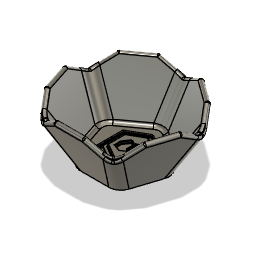
GB - Porta D12 (Autodesk Fusion 360 design; units mm, degrees)
Autodesk Fusion 360 part; units mm, degrees
note: some values were not read from the file. Chosen so that the rebuilt part matches the saved one: which bodies a step acts on; which face or edge a step refers to. Set by a fixed rule: which sketch regions a step uses.
sketch "Sketch1" plane through (0, 0, 0) normal (0, 1, 0) x (1, 0, 0)
  line L0 (-5, -6.8819) -> (5, -6.8819)
  line L1 (5, -6.8819) -> (8.0902, 2.6287)
  line L2 (8.0902, 2.6287) -> (0, 8.5065)
  line L3 (0, 8.5065) -> (-8.0902, 2.6287)
  line L4 (-8.0902, 2.6287) -> (-5, -6.8819)
  dimension "d1" = 10
  constraint horizontal L0
  measures "d1" distance of L0.start L0.end
ref_plane "WorkPlane1" through (0, 0, 6.8819) normal (0, -0.447213, 0.894428) x (1, 0, 0)
ref_plane "WorkPlane2" through (-6.5451, 0, 2.1266) normal (-0.850651, -0.447213, 0.276393) x (0.309017, 0, 0.951057)
ref_plane "WorkPlane3" through (-4.0451, 0, -5.5676) normal (0.525731, 0.447213, 0.723607) x (-0.809017, 0, 0.587785)
ref_plane "WorkPlane4" through (4.0451, 0, -5.5676) normal (-0.525731, 0.447213, 0.723607) x (-0.809017, 0, -0.587785)
ref_plane "WorkPlane5" through (6.5451, 0, 2.1266) normal (0.850651, -0.447213, 0.276393) x (0.309017, 0, -0.951057)
sketch "Sketch2" plane through (15, -2.7528, 5.5055) normal (0, -0.447213, 0.894428) x (1, 0, 0)
  line L0 (-10, 3.0777) -> (-6.9098, 12.5882)
  line L1 (-6.9098, 12.5882) -> (-15, 18.4661)
  line L2 (-15, 18.4661) -> (-23.0902, 12.5882)
  line L3 (-23.0902, 12.5882) -> (-20, 3.0777)
  line L4 (-20, 3.0777) -> (-10, 3.0777)
  point P0 (-15, 9.9596)
  point P1 (-10, 3.0777)
  point P2 (-20, 3.0777)
  constraint coincident L0.start L4.end
  constraint coincident P2 L3.end
sketch "Sketch3" plane through (18.1631, 8.6599, -19.618) normal (0.850651, -0.447213, 0.276393) x (0.309017, 0, -0.951057)
  line L0 (-19.2705, -9.6821) -> (-16.1803, -0.1715)
  line L1 (-16.1803, -0.1715) -> (-24.2705, 5.7064)
  line L2 (-24.2705, 5.7064) -> (-32.3607, -0.1715)
  line L3 (-32.3607, -0.1715) -> (-29.2705, -9.6821)
  line L4 (-29.2705, -9.6821) -> (-19.2705, -9.6821)
  point P0 (-24.2705, -2.8002)
  point P1 (-19.2705, -9.6821)
  point P2 (-29.2705, -9.6821)
  constraint coincident P2 L3.end
  constraint coincident L0.start L4.end
sketch "Sketch4" plane through (8.6631, 15.7133, -11.9237) normal (-0.525731, 0.447213, 0.723607) x (-0.809017, 0, -0.587785)
  line L0 (5, 17.568) -> (-5, 17.568)
  line L1 (-5, 17.568) -> (-8.0902, 8.0574)
  line L2 (-8.0902, 8.0574) -> (0, 2.1796)
  line L3 (0, 2.1796) -> (8.0902, 8.0574)
  line L4 (8.0902, 8.0574) -> (5, 17.568)
  point P0 (0, 10.6861)
  point P1 (5, 17.568)
  point P2 (-5, 17.568)
  constraint coincident L0.end L1.start
  constraint coincident L0.start L4.end
sketch "Sketch5" plane through (13.0451, 8.6599, -23.3364) normal (0.525731, 0.447213, 0.723607) x (-0.809017, 0, 0.587785)
  line L0 (29.2705, 9.6821) -> (19.2705, 9.6821)
  line L1 (19.2705, 9.6821) -> (16.1803, 0.1715)
  line L2 (16.1803, 0.1715) -> (24.2705, -5.7064)
  line L3 (24.2705, -5.7064) -> (32.3607, 0.1715)
  line L4 (32.3607, 0.1715) -> (29.2705, 9.6821)
  point P0 (24.2705, 2.8002)
  point P1 (29.2705, 9.6821)
  point P2 (19.2705, 9.6821)
  constraint coincident L0.end L1.start
  constraint coincident L0.start L4.end
sketch "Sketch6" plane through (-9.8713, -2.7528, -12.5645) normal (-0.850651, -0.447213, 0.276393) x (0.309017, 0, 0.951057)
  line L0 (20, 3.0777) -> (23.0902, 12.5882)
  line L1 (23.0902, 12.5882) -> (15, 18.4661)
  line L2 (15, 18.4661) -> (6.9098, 12.5882)
  line L3 (6.9098, 12.5882) -> (10, 3.0777)
  line L4 (10, 3.0777) -> (20, 3.0777)
  point P0 (15, 9.9596)
  point P1 (10, 3.0777)
  point P2 (20, 3.0777)
  constraint coincident P1 L3.end
  constraint coincident P2 L0.start
extrude "Extrude2" add sketch "Sketch1" along normal blind 2 makes body 1
extrude "Extrude3" add sketch "Sketch6" against normal blind 1 bodies 1
extrude "Extrude4" add sketch "Sketch2" against normal blind 1 bodies 1
extrude "Extrude5" add sketch "Sketch3" against normal blind 1 bodies 1
extrude "Extrude6" add sketch "Sketch4" along normal blind 1 bodies 1
extrude "Extrude7" add sketch "Sketch5" along normal blind 1 bodies 1
ref_plane "WorkPlane9" through (0, 12, 0) normal (0, 1, 0) x (0, 0, 1)
split "Split1" by plane through (0, 12, 0) normal (0, 1, 0) bodies 1 makes body 2 at (-7.1312, 12.737, -9.8153) makes body 3 at (-11.5386, 12.737, 3.7491) makes body 4 at (0, 12.737, 12.1324) makes body 5 at (7.1312, 12.737, -9.8153) makes body 6 at (11.5386, 12.737, 3.7491)
delete_body "RemoveBody1" bodies 5
delete_body "RemoveBody2" bodies 4
delete_body "RemoveBody3" bodies 6
delete_body "RemoveBody4" bodies 3
delete_body "RemoveBody5" bodies 2
fillet "Fillet2" radius 3 10 edges at (-6.5451, 4.2533, 9.0085) (-10.5902, 4.2533, -3.441) (0, 4.2533, -11.1352) (10.5902, 4.2533, -3.441) (6.5451, 4.2533, 9.0085) (0, 5.6477, -10.615) (6.2393, 5.6477, 8.5877) (-6.2393, 5.6477, 8.5877) (10.0955, 5.6477, -3.2802) (-10.0955, 5.6477, -3.2802) on bodies 1
fillet "Fillet6" radius 1 10 edges at (-3.9757, 2, -5.4721) (-7.3625, 2, -2.3922) (0, 2, -7.7414) (-6.4328, 2, 2.0902) (3.9757, 2, -5.4721) (-4.5503, 2, 6.2629) (7.3625, 2, -2.3922) (0, 2, 6.7639) (6.4328, 2, 2.0902) (4.5503, 2, 6.2629) on bodies 1
sketch "Sketch8" plane through (0, 2, 0) normal (0, 1, 0) x (-1, 0, 0)
  line L0 (0, -4.7528) -> (3.25, -2.8764)
  line L1 (3.25, -2.8764) -> (3.25, 0.8764)
  line L2 (3.25, 0.8764) -> (0, 2.7528)
  line L3 (0, 2.7528) -> (-3.25, 0.8764)
  line L4 (-3.25, 0.8764) -> (-3.25, -2.8764)
  line L5 (-3.25, -2.8764) -> (0, -4.7528)
  line L6 (0, 0) -> (0, -1)
  line L7 (0, 3.6188) -> (-3.25, 1.7424)
  line L8 (-4, 1.3094) -> (-4, -3.3094)
  line L9 (-4, -3.3094) -> (0, -5.6188)
  line L10 (0, -5.6188) -> (4, -3.3094)
  line L11 (4, -3.3094) -> (4, 1.3094)
  line L12 (3.25, 1.7424) -> (0, 3.6188)
  line L13 (-4, 1.3094) -> (-4, 2.3094)
  line L14 (4, 1.3094) -> (4, 2.3094)
  line L15 (-3.25, 2.7424) -> (0, 4.6188)
  line L16 (0, 3.6188) -> (0, 4.6188)
  line L17 (-4, 2.3094) -> (-4, 3.0594)
  line L18 (0, 4.6188) -> (0, 5.3688)
  line L19 (-4, 3.0594) -> (0, 5.3688)
  line L20 (-3.25, 1.7424) -> (-3.25, 2.7424)
  line L21 (4, 2.3094) -> (0, 4.6188)
  line L22 (3.25, 1.7424) -> (3.25, 2.7424)
  line L23 (0, 5.3688) -> (4, 3.0594)
  line L24 (4, 3.0594) -> (4, 2.3094)
  line L25 (0, 0) -> (0, 3.6188)
  line L26 (0, 4.6188) -> (0, 5.3688)
  line L27 (0, 3.6188) -> (0, 4.6188)
  line L28 (-3.25, 1.7424) -> (-4, 1.3094)
  line L29 (-4, 2.3094) -> (-3.25, 2.7424)
  line L30 (4, 1.3094) -> (3.25, 1.7424)
  point P0 (0, -1)
  point P1 (0, -1)
  dimension "d35" = 1
  dimension "d37" = 1
  dimension "d40" = 0.75
  dimension "d43" = 3.25
  dimension "d44" = 4
  constraint coincident L6.start L25.start
  constraint coincident P1 P0
  constraint parallel L8 L13
  constraint parallel L11 L14
  constraint parallel L13 L17
  constraint parallel L16 L18
  constraint collinear L4 L20
  constraint coincident L21 L22.end
  constraint parallel L6 L25
  constraint collinear L1 L22
  constraint collinear L11 L24
  constraint vertical L25
  constraint parallel L2 L12
  constraint parallel L12 L21
  constraint equal L13 L14
  constraint equal L17 L24
  constraint vertical L11
  constraint parallel L2 L30
  constraint equal L13 L27
  constraint equal L17 L18
  measures "d35" distance of L6.start P1
  measures "d37" distance of L8.start L13.end
  measures "d40" distance of L13.end L17.end
  measures "d43" distance of P1 L4
  measures "d44" distance of P1 L8
sketch "Sketch9" plane through (0, 2, 0) normal (0, 1, 0) x (-1, 0, 0)
  line L0 (3.1655, 6.1458) -> (-3.1655, 6.1458)
  line L1 (-4.8668, 4.9098) -> (-6.8232, -1.1114)
  line L2 (-6.1734, -3.1114) -> (-1.0515, -6.8327)
  line L3 (1.0515, -6.8327) -> (6.1734, -3.1114)
  line L4 (6.8232, -1.1114) -> (4.8668, 4.9098)
  ellipse E0 centre (4.5962, -1.4934) end of major axis (6.8323, -2.2199) minor radius 2 (6.1734, -3.1114) -> (6.8232, -1.1114) ccw construction
  ellipse E1 centre (2.8406, 3.9098) end of major axis (4.2226, 5.8119) minor radius 2 (4.8668, 4.9098) -> (3.1655, 6.1458) ccw construction
  ellipse E2 centre (-2.8406, 3.9098) end of major axis (-4.2226, 5.8119) minor radius 2 (-3.1655, 6.1458) -> (-4.8668, 4.9098) ccw construction
  ellipse E3 centre (-4.5962, -1.4934) end of major axis (-6.8323, -2.2199) minor radius 2 (-6.8232, -1.1114) -> (-6.1734, -3.1114) ccw construction
  ellipse E4 centre (0, -4.8327) end of major axis (0, -7.1839) minor radius 2 (-1.0515, -6.8327) -> (1.0515, -6.8327) ccw construction
  line L5 (-2.5118, -0.3911) -> (-2.3485, -1.8376)
  line L6 (-2.3485, -1.8376) -> (-1.4619, -2.8642)
  line L7 (-1.4619, -2.8642) -> (0.0888, -2.1176)
  line L8 (0.0888, -2.1176) -> (0.0888, -0.5078)
  line L9 (0.0888, -0.5078) -> (-0.8554, 0.3088)
  line L10 (-0.8554, 0.3088) -> (-2.5118, -0.3911)
  line L11 (0.3403, -1.9543) -> (1.2969, -2.4428)
  line L12 (1.2969, -2.4428) -> (2.2301, -1.0662)
  line L13 (2.2301, -1.0662) -> (2.2301, 0.217)
  line L14 (2.2301, 0.217) -> (0.7836, 0.7535)
  line L15 (0.7836, 0.7535) -> (-0.213, 0.045)
  line L16 (-0.213, 0.045) -> (0.3403, -0.413)
  line L17 (0.3403, -0.413) -> (0.3403, -1.9543)
extrude "Extrude8" cut sketch "Sketch8" sketch "Sketch9" against normal blind 0.5 contours L7 L8 L9 L10 L11 L12 L28 L30 | L13 L20 L28 L29 | L14 L21 L22 L30 | L15 L17 L18 L19 L26 L29 | L18 L21 L23 L24 L26 of sketch 2 bodies 1
fillet "Fillet8" radius 0.1 31 edges at (2, 1.5, -4.4641) (-2, 1.5, -4.4641) (-4, 1.5, -0.125) (-2, 1.5, 4.2141) (2, 1.5, 4.2141) (4, 1.5, -0.125) (1.625, 1.5, 3.6806) (-1.625, 1.5, 3.6806) (-3.25, 1.5, 2.2424) (-1.625, 1.5, 2.6806) (1.625, 1.5, 2.6806) (3.25, 1.5, 2.2424) (1.625, 1.5, -3.8146) (3.25, 1.5, -1) (1.625, 1.5, 1.8146) (-1.625, 1.5, 1.8146) (-3.25, 1.5, -1) (-1.625, 1.5, -3.8146) (-0.3403, 1.5, -1.1836) (-0.8186, 1.5, -2.1985) (-1.7635, 1.5, -1.7545) (-2.2301, 1.5, -0.4246) (-1.5069, 1.5, 0.4852) (-0.2853, 1.5, 0.3993) (-0.0637, 1.5, -0.184) (1.6836, 1.5, -0.0412) (2.4301, 1.5, -1.1144) (1.9052, 1.5, -2.3509) (0.6866, 1.5, -2.4909) (-0.0888, 1.5, -1.3127) (0.3833, 1.5, -0.0995) on bodies 1
fillet "Fillet9" radius 0.15 18 edges at (2, 2, 4.2141) (4, 2, -0.125) (1.625, 2, 3.6806) (1.625, 2, 2.6806) (3.25, 2, 2.2424) (-1.625, 2, 2.6806) (-1.625, 2, 3.6806) (-2, 2, 4.2141) (-4, 2, -0.125) (-1.625, 2, 1.8146) (-3.25, 2, 2.2424) (-2, 2, -4.4641) (-1.625, 2, -3.8146) (2, 2, -4.4641) (1.625, 2, -3.8146) (3.25, 2, -1) (-3.25, 2, -1) (1.625, 2, 1.8146) on bodies 1
fillet "Fillet10" radius 0.1 13 edges at (0.6866, 2, -2.4909) (1.9052, 2, -2.3509) (2.4301, 2, -1.1144) (1.6836, 2, -0.0412) (0.3833, 2, -0.0995) (-0.2853, 2, 0.3993) (-0.3403, 2, -1.1836) (-1.5069, 2, 0.4852) (-0.0637, 2, -0.184) (-2.2301, 2, -0.4246) (-1.7635, 2, -1.7545) (-0.8186, 2, -2.1985) (-0.0888, 2, -1.3127) on bodies 1
fillet "Fillet12" radius 0.5 65 edges at (-10.466, 11.1601, -6.4179) (-6.9146, 12, -9.5172) (-2.8696, 11.1601, -11.937) (-11.6357, 9.9182, -4.6427) (-12.1424, 9.9182, -3.0833) (0.8198, 9.9182, -12.5009) (-0.8198, 9.9182, -12.5009) (-12.2395, 11.1601, -0.9596) (-11.1881, 12, 3.6352) (-9.3379, 11.1601, 7.9705) (10.466, 11.1601, -6.4179) (6.9146, 12, -9.5172) (2.8696, 11.1601, -11.937) (-6.6846, 9.9182, 10.5953) (-8.0111, 9.9182, 9.6316) (12.1424, 9.9182, -3.0833) (11.6357, 9.9182, -4.6427) (-4.6948, 11.1601, 11.3439) (0, 12, 11.7639) (4.6948, 11.1601, 11.3439) (12.2395, 11.1601, -0.9596) (11.1881, 12, 3.6352) (9.3379, 11.1601, 7.9705) (8.0111, 9.9182, 9.6316) (6.6846, 9.9182, 10.5953) (-12.2837, 9.2544, -3.9912) (-12.4864, 9.1293, -4.9191) (-10.9415, 10.7657, -7.2106) (-9.7175, 12, -8.1718) (-4.769, 12, -11.7671) (-7.5718, 12, -10.4217) (0, 9.2544, -12.9159) (-0.8198, 9.1293, -13.3953) (-3.4766, 10.7657, -12.6342) (-12.993, 9.1293, -3.3597) (-13.0902, 10.7657, -0.5978) (-12.6648, 12, 0.8993) (0.8198, 9.1293, -13.3953) (3.4766, 10.7657, -12.6342) (4.769, 12, -11.7671) (-12.2514, 12, 3.9807) (-10.7747, 12, 6.7166) (-7.5917, 9.2544, 10.4491) (-8.5368, 9.1293, 10.3552) (-10.2388, 10.7657, 8.1778) (12.2837, 9.2544, -3.9912) (12.4864, 9.1293, -4.9191) (10.9415, 10.7657, -7.2106) (9.7175, 12, -8.1718) (7.5718, 12, -10.4217) (-7.2103, 9.1293, 11.3189) (-4.6136, 10.7657, 12.2648) (-3.0583, 12, 12.3229) (12.993, 9.1293, -3.3597) (13.0902, 10.7657, -0.5978) (12.6648, 12, 0.8993) (0, 12, 12.8819) (3.0583, 12, 12.3229) (7.5917, 9.2544, 10.4491) (7.2103, 9.1293, 11.3189) (4.6136, 10.7657, 12.2648) (12.2514, 12, 3.9807) (10.7747, 12, 6.7166) (8.5368, 9.1293, 10.3552) (10.2388, 10.7657, 8.1778) on bodies 1
sketch "Sketch10" plane through (0, 0, 0) normal (0, -1, 0) x (1, 0, 0)
  ellipse E0 centre (2.5631, 3.5278) end of major axis (4.6361, 6.381) minor radius 3 (5.6024, 5.0278) -> (3.0505, 6.8819) ccw
  line L0 (3.0505, 6.8819) -> (-3.0505, 6.8819)
  ellipse E1 centre (-2.5631, 3.5278) end of major axis (-4.6361, 6.381) minor radius 3 (-3.0505, 6.8819) -> (-5.6024, 5.0278) ccw
  line L1 (-5.6024, 5.0278) -> (-7.4877, -0.7746)
  ellipse E2 centre (-4.1472, -1.3475) end of major axis (-7.5013, -2.4373) minor radius 3 (-7.4877, -0.7746) -> (-6.513, -3.7746) ccw
  line L2 (-6.513, -3.7746) -> (-1.5772, -7.3606)
  ellipse E3 centre (0, -4.3606) end of major axis (0, -7.8873) minor radius 3 (-1.5772, -7.3606) -> (1.5772, -7.3606) ccw
  line L3 (1.5772, -7.3606) -> (6.513, -3.7746)
  ellipse E4 centre (4.1472, -1.3475) end of major axis (7.5013, -2.4373) minor radius 3 (6.513, -3.7746) -> (7.4877, -0.7746) ccw
  line L4 (7.4877, -0.7746) -> (5.6024, 5.0278)
  line L5 (0, 4) -> (-3.4641, -2)
  line L6 (-3.4641, -2) -> (3.4641, -2)
  line L7 (3.4641, -2) -> (0, 4)
  dimension "d50" = 2
  constraint horizontal L6
  measures "d50" distance of origin L7
extrude "Extrude9" cut sketch "Sketch10" against normal blind 1 contours L5 L6 L7 bodies 1
equation "d1 = lado"
equation "lado = 10 mm"
named bodies: "PortaD12", "PortaD12 (1)", "PortaD12 (2)", "PortaD12 (3)", "PortaD12 (4)", "PortaD12 (5)"
